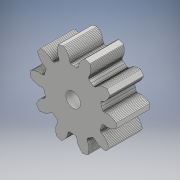
# Autodesk Inventor part: Engranajes PEQUENO final 2017
Saved by Autodesk Inventor 2019 (Build 230136000, 136)
## iProperties
Created: 2017-09-25
Part Number: Engranajes PEQUENO final 2017
Material: Generic
Document SubType Name: Modeling
Designer: ANDRES
Density: 1 g/cm^3
Appearance: Default
Author: ANDRES
## iProperties of the stored document Engranajes PEQUENO final 2017_3DPrint.ipt
Created: 2017-09-25
Part Number: Engranajes PEQUENO final 2017_3DPrint
Material: Generic
Document SubType Name: Modeling
Designer: ANDRES
Density: 1 g/cm^3
Appearance: Default
Author: ANDRES
Autodesk Inventor part; units mm, degrees
ref_plane "YZ Plane" through (0, 0, 0) normal (1, 0, 0) x (0, 1, 0)
ref_plane "XZ Plane" through (0, 0, 0) normal (0, 1, 0) x (-1, 0, 0)
ref_plane "XY Plane" through (0, 0, 0) normal (0, 0, 1) x (1, 0, 0)
sketch "Sketch1" plane through (0, 0, 0) normal (0, 1, 0) x (-1, 0, 0)
  line L0 (1.2686, 3.1496) -> (1.234, 3.2065)
  line L1 (1.234, 3.2065) -> (1.2093, 3.2258)
  line L2 (1.2093, 3.2258) -> (1.1862, 3.2384)
  line L3 (1.1862, 3.2384) -> (1.1641, 3.2475)
  line L4 (1.1641, 3.2475) -> (1.1425, 3.2542)
  line L5 (1.1425, 3.2542) -> (1.1214, 3.259)
  line L6 (1.1214, 3.259) -> (1.08, 3.2647)
  line L7 (1.08, 3.2647) -> (1.0396, 3.2662)
  line L8 (1.0396, 3.2662) -> (0.9998, 3.2645)
  line L9 (0.9998, 3.2645) -> (0.9218, 3.2535)
  line L10 (0.9218, 3.2535) -> (0.8454, 3.2341)
  line L11 (0.8454, 3.2341) -> (0.7662, 3.2294)
  line L12 (0.7662, 3.2294) -> (0.6848, 3.2361)
  line L13 (0.6848, 3.2361) -> (0.6022, 3.2499)
  line L14 (0.6022, 3.2499) -> (0.5189, 3.27)
  line L15 (0.5189, 3.27) -> (0.435, 3.2958)
  line L16 (0.435, 3.2958) -> (0.3507, 3.3269)
  line L17 (0.3507, 3.3269) -> (0.2664, 3.3631)
  line L18 (0.2664, 3.3631) -> (0.182, 3.4043)
  line L19 (0.182, 3.4043) -> (0.0978, 3.4503)
  line L20 (0.0978, 3.4503) -> (0.0141, 3.5011)
  line L21 (0.0141, 3.5011) -> (0.0024, 3.9651)
  line L22 (0.0024, 3.9651) -> (0.0835, 4.02)
  line L23 (0.0835, 4.02) -> (0.1653, 4.0702)
  line L24 (0.1653, 4.0702) -> (0.2474, 4.1155)
  line L25 (0.2474, 4.1155) -> (0.3299, 4.156)
  line L26 (0.3299, 4.156) -> (0.4125, 4.1913)
  line L27 (0.4125, 4.1913) -> (0.495, 4.2212)
  line L28 (0.495, 4.2212) -> (0.5772, 4.2455)
  line L29 (0.5772, 4.2455) -> (0.659, 4.2635)
  line L30 (0.659, 4.2635) -> (0.7399, 4.2742)
  line L31 (0.7399, 4.2742) -> (0.8193, 4.2735)
  line L32 (0.8193, 4.2735) -> (0.8965, 4.258)
  line L33 (0.8965, 4.258) -> (0.975, 4.2509)
  line L34 (0.975, 4.2509) -> (1.0148, 4.2512)
  line L35 (1.0148, 4.2512) -> (1.0551, 4.2547)
  line L36 (1.0551, 4.2547) -> (1.0962, 4.2625)
  line L37 (1.0962, 4.2625) -> (1.117, 4.2684)
  line L38 (1.117, 4.2684) -> (1.1382, 4.2761)
  line L39 (1.1382, 4.2761) -> (1.1599, 4.2863)
  line L40 (1.1599, 4.2863) -> (1.1823, 4.3001)
  line L41 (1.1823, 4.3001) -> (1.206, 4.3206)
  line L42 (1.206, 4.3206) -> (1.2377, 4.3791)
  line L43 (1.2377, 4.3791) -> (1.2899, 4.5842)
  line L44 (1.2899, 4.5842) -> (1.3582, 4.7844)
  line L45 (1.3582, 4.7844) -> (1.3636, 4.8508)
  line L46 (1.3636, 4.8508) -> (1.355, 4.8809)
  line L47 (1.355, 4.8809) -> (1.3438, 4.9047)
  line L48 (1.3438, 4.9047) -> (1.3312, 4.9251)
  line L49 (1.3312, 4.9251) -> (1.3177, 4.9431)
  line L50 (1.3177, 4.9431) -> (1.3034, 4.9595)
  line L51 (1.3034, 4.9595) -> (1.2733, 4.9884)
  line L52 (1.2733, 4.9884) -> (1.2415, 5.0134)
  line L53 (1.2415, 5.0134) -> (1.2083, 5.0354)
  line L54 (1.2083, 5.0354) -> (1.1387, 5.0723)
  line L55 (1.1387, 5.0723) -> (1.0655, 5.1015)
  line L56 (1.0655, 5.1015) -> (0.9986, 5.1443)
  line L57 (0.9986, 5.1443) -> (0.9367, 5.1975)
  line L58 (0.9367, 5.1975) -> (0.8781, 5.2573)
  line L59 (0.8781, 5.2573) -> (0.8225, 5.3225)
  line L60 (0.8225, 5.3225) -> (0.7697, 5.3927)
  line L61 (0.7697, 5.3927) -> (0.7198, 5.4674)
  line L62 (0.7198, 5.4674) -> (0.6729, 5.5463)
  line L63 (0.6729, 5.5463) -> (0.6288, 5.6292)
  line L64 (0.6288, 5.6292) -> (0.5878, 5.7159)
  line L65 (0.5878, 5.7159) -> (0.5499, 5.8062)
  line L66 (0.5499, 5.8062) -> (0.8132, 6.1884)
  line L67 (0.8132, 6.1884) -> (0.9111, 6.1852)
  line L68 (0.9111, 6.1852) -> (1.0067, 6.1777)
  line L69 (1.0067, 6.1777) -> (1.0998, 6.1661)
  line L70 (1.0998, 6.1661) -> (1.1903, 6.1504)
  line L71 (1.1903, 6.1504) -> (1.2779, 6.1304)
  line L72 (1.2779, 6.1304) -> (1.3622, 6.1061)
  line L73 (1.3622, 6.1061) -> (1.443, 6.0774)
  line L74 (1.443, 6.0774) -> (1.5197, 6.0439)
  line L75 (1.5197, 6.0439) -> (1.5915, 6.005)
  line L76 (1.5915, 6.005) -> (1.6553, 5.9578)
  line L77 (1.6553, 5.9578) -> (1.7087, 5.8998)
  line L78 (1.7087, 5.8998) -> (1.768, 5.848)
  line L79 (1.768, 5.848) -> (1.8004, 5.8248)
  line L80 (1.8004, 5.8248) -> (1.8351, 5.804)
  line L81 (1.8351, 5.804) -> (1.8728, 5.7861)
  line L82 (1.8728, 5.7861) -> (1.8932, 5.7786)
  line L83 (1.8932, 5.7786) -> (1.9149, 5.7724)
  line L84 (1.9149, 5.7724) -> (1.9384, 5.7679)
  line L85 (1.9384, 5.7679) -> (1.9646, 5.766)
  line L86 (1.9646, 5.766) -> (1.9959, 5.7686)
  line L87 (1.9959, 5.7686) -> (2.0559, 5.7973)
  line L88 (2.0559, 5.7973) -> (2.2187, 5.9324)
  line L89 (2.2187, 5.9324) -> (2.3916, 6.0542)
  line L90 (2.3916, 6.0542) -> (2.435, 6.1047)
  line L91 (2.435, 6.1047) -> (2.4457, 6.1342)
  line L92 (2.4457, 6.1342) -> (2.4506, 6.1601)
  line L93 (2.4506, 6.1601) -> (2.4524, 6.1839)
  line L94 (2.4524, 6.1839) -> (2.4521, 6.2065)
  line L95 (2.4521, 6.2065) -> (2.4502, 6.2281)
  line L96 (2.4502, 6.2281) -> (2.4428, 6.2692)
  line L97 (2.4428, 6.2692) -> (2.4318, 6.3081)
  line L98 (2.4318, 6.3081) -> (2.4177, 6.3454)
  line L99 (2.4177, 6.3454) -> (2.3831, 6.4162)
  line L100 (2.3831, 6.4162) -> (2.3411, 6.4828)
  line L101 (2.3411, 6.4828) -> (2.3122, 6.5568)
  line L102 (2.3122, 6.5568) -> (2.2933, 6.6362)
  line L103 (2.2933, 6.6362) -> (2.281, 6.719)
  line L104 (2.281, 6.719) -> (2.2743, 6.8045)
  line L105 (2.2743, 6.8045) -> (2.2728, 6.8923)
  line L106 (2.2728, 6.8923) -> (2.2764, 6.982)
  line L107 (2.2764, 6.982) -> (2.2848, 7.0734)
  line L108 (2.2848, 7.0734) -> (2.2979, 7.1664)
  line L109 (2.2979, 7.1664) -> (2.3155, 7.2606)
  line L110 (2.3155, 7.2606) -> (2.3379, 7.356)
  line L111 (2.3379, 7.356) -> (2.7756, 7.5106)
  line L112 (2.7756, 7.5106) -> (2.8529, 7.4504)
  line L113 (2.8529, 7.4504) -> (2.9259, 7.3882)
  line L114 (2.9259, 7.3882) -> (2.9944, 7.3241)
  line L115 (2.9944, 7.3241) -> (3.0584, 7.2582)
  line L116 (3.0584, 7.2582) -> (3.1175, 7.1906)
  line L117 (3.1175, 7.1906) -> (3.1715, 7.1214)
  line L118 (3.1715, 7.1214) -> (3.22, 7.0507)
  line L119 (3.22, 7.0507) -> (3.2624, 6.9785)
  line L120 (3.2624, 6.9785) -> (3.2976, 6.9048)
  line L121 (3.2976, 6.9048) -> (3.3215, 6.8291)
  line L122 (3.3215, 6.8291) -> (3.3307, 6.7508)
  line L123 (3.3307, 6.7508) -> (3.3482, 6.674)
  line L124 (3.3482, 6.674) -> (3.3608, 6.6362)
  line L125 (3.3608, 6.6362) -> (3.3766, 6.599)
  line L126 (3.3766, 6.599) -> (3.3966, 6.5624)
  line L127 (3.3966, 6.5624) -> (3.4087, 6.5443)
  line L128 (3.4087, 6.5443) -> (3.4226, 6.5267)
  line L129 (3.4226, 6.5267) -> (3.439, 6.5092)
  line L130 (3.439, 6.5092) -> (3.459, 6.4922)
  line L131 (3.459, 6.4922) -> (3.4859, 6.476)
  line L132 (3.4859, 6.476) -> (3.5513, 6.4639)
  line L133 (3.5513, 6.4639) -> (3.7625, 6.4776)
  line L134 (3.7625, 6.4776) -> (3.974, 6.4746)
  line L135 (3.974, 6.4746) -> (4.0388, 6.49)
  line L136 (4.0388, 6.49) -> (4.0648, 6.5075)
  line L137 (4.0648, 6.5075) -> (4.084, 6.5255)
  line L138 (4.084, 6.5255) -> (4.0994, 6.5438)
  line L139 (4.0994, 6.5438) -> (4.1124, 6.5622)
  line L140 (4.1124, 6.5622) -> (4.1236, 6.5808)
  line L141 (4.1236, 6.5808) -> (4.1417, 6.6184)
  line L142 (4.1417, 6.6184) -> (4.1557, 6.6564)
  line L143 (4.1557, 6.6564) -> (4.1664, 6.6948)
  line L144 (4.1664, 6.6948) -> (4.18, 6.7724)
  line L145 (4.18, 6.7724) -> (4.1851, 6.851)
  line L146 (4.1851, 6.851) -> (4.2052, 6.9278)
  line L147 (4.2052, 6.9278) -> (4.2366, 7.0032)
  line L148 (4.2366, 7.0032) -> (4.2753, 7.0774)
  line L149 (4.2753, 7.0774) -> (4.3201, 7.1504)
  line L150 (4.3201, 7.1504) -> (4.3705, 7.2223)
  line L151 (4.3705, 7.2223) -> (4.4262, 7.2928)
  line L152 (4.4262, 7.2928) -> (4.4867, 7.3619)
  line L153 (4.4867, 7.3619) -> (4.5519, 7.4295)
  line L154 (4.5519, 7.4295) -> (4.6217, 7.4952)
  line L155 (4.6217, 7.4952) -> (4.6958, 7.5591)
  line L156 (4.6958, 7.5591) -> (5.1408, 7.4269)
  line L157 (5.1408, 7.4269) -> (5.1679, 7.3327)
  line L158 (5.1679, 7.3327) -> (5.1904, 7.2395)
  line L159 (5.1904, 7.2395) -> (5.208, 7.1473)
  line L160 (5.208, 7.1473) -> (5.221, 7.0564)
  line L161 (5.221, 7.0564) -> (5.2292, 6.967)
  line L162 (5.2292, 6.967) -> (5.2321, 6.8792)
  line L163 (5.2321, 6.8792) -> (5.2298, 6.7935)
  line L164 (5.2298, 6.7935) -> (5.2216, 6.7102)
  line L165 (5.2216, 6.7102) -> (5.2068, 6.63)
  line L166 (5.2068, 6.63) -> (5.1816, 6.5546)
  line L167 (5.1816, 6.5546) -> (5.143, 6.486)
  line L168 (5.143, 6.486) -> (5.112, 6.4136)
  line L169 (5.112, 6.4136) -> (5.1001, 6.3756)
  line L170 (5.1001, 6.3756) -> (5.091, 6.3362)
  line L171 (5.091, 6.3362) -> (5.0857, 6.2948)
  line L172 (5.0857, 6.2948) -> (5.0849, 6.2731)
  line L173 (5.0849, 6.2731) -> (5.0857, 6.2505)
  line L174 (5.0857, 6.2505) -> (5.0887, 6.2268)
  line L175 (5.0887, 6.2268) -> (5.0949, 6.2012)
  line L176 (5.0949, 6.2012) -> (5.1071, 6.1723)
  line L177 (5.1071, 6.1723) -> (5.1529, 6.124)
  line L178 (5.1529, 6.124) -> (5.3318, 6.0111)
  line L179 (5.3318, 6.0111) -> (5.5011, 5.8842)
  line L180 (5.5011, 5.8842) -> (5.5625, 5.8587)
  line L181 (5.5625, 5.8587) -> (5.5939, 5.8576)
  line L182 (5.5939, 5.8576) -> (5.62, 5.8609)
  line L183 (5.62, 5.8609) -> (5.6433, 5.8666)
  line L184 (5.6433, 5.8666) -> (5.6646, 5.8738)
  line L185 (5.6646, 5.8738) -> (5.6846, 5.8823)
  line L186 (5.6846, 5.8823) -> (5.7213, 5.9021)
  line L187 (5.7213, 5.9021) -> (5.755, 5.9246)
  line L188 (5.755, 5.9246) -> (5.7861, 5.9494)
  line L189 (5.7861, 5.9494) -> (5.8428, 6.0042)
  line L190 (5.8428, 6.0042) -> (5.8932, 6.0647)
  line L191 (5.8932, 6.0647) -> (5.9545, 6.1151)
  line L192 (5.9545, 6.1151) -> (6.0243, 6.1575)
  line L193 (6.0243, 6.1575) -> (6.0992, 6.1948)
  line L194 (6.0992, 6.1948) -> (6.1784, 6.2277)
  line L195 (6.1784, 6.2277) -> (6.2615, 6.2562)
  line L196 (6.2615, 6.2562) -> (6.3479, 6.2805)
  line L197 (6.3479, 6.2805) -> (6.4375, 6.3008)
  line L198 (6.4375, 6.3008) -> (6.5299, 6.3171)
  line L199 (6.5299, 6.3171) -> (6.6251, 6.3293)
  line L200 (6.6251, 6.3293) -> (6.7227, 6.3375)
  line L201 (6.7227, 6.3375) -> (7.0048, 5.969)
  line L202 (7.0048, 5.969) -> (6.9715, 5.8769)
  line L203 (6.9715, 5.8769) -> (6.935, 5.7883)
  line L204 (6.935, 5.7883) -> (6.8951, 5.7033)
  line L205 (6.8951, 5.7033) -> (6.8522, 5.6221)
  line L206 (6.8522, 5.6221) -> (6.8061, 5.5449)
  line L207 (6.8061, 5.5449) -> (6.757, 5.4722)
  line L208 (6.757, 5.4722) -> (6.7047, 5.4043)
  line L209 (6.7047, 5.4043) -> (6.6492, 5.3416)
  line L210 (6.6492, 5.3416) -> (6.59, 5.2854)
  line L211 (6.59, 5.2854) -> (6.5253, 5.2393)
  line L212 (6.5253, 5.2393) -> (6.4538, 5.2064)
  line L213 (6.4538, 5.2064) -> (6.3862, 5.1661)
  line L214 (6.3862, 5.1661) -> (6.3541, 5.1424)
  line L215 (6.3541, 5.1424) -> (6.3236, 5.1158)
  line L216 (6.3236, 5.1158) -> (6.295, 5.0855)
  line L217 (6.295, 5.0855) -> (6.2816, 5.0684)
  line L218 (6.2816, 5.0684) -> (6.269, 5.0497)
  line L219 (6.269, 5.0497) -> (6.2574, 5.0287)
  line L220 (6.2574, 5.0287) -> (6.2474, 5.0044)
  line L221 (6.2474, 5.0044) -> (6.2403, 4.9739)
  line L222 (6.2403, 4.9739) -> (6.249, 4.9079)
  line L223 (6.249, 4.9079) -> (6.3273, 4.7113)
  line L224 (6.3273, 4.7113) -> (6.3897, 4.5092)
  line L225 (6.3897, 4.5092) -> (6.4244, 4.4523)
  line L226 (6.4244, 4.4523) -> (6.4491, 4.433)
  line L227 (6.4491, 4.433) -> (6.4722, 4.4203)
  line L228 (6.4722, 4.4203) -> (6.4943, 4.4113)
  line L229 (6.4943, 4.4113) -> (6.5159, 4.4046)
  line L230 (6.5159, 4.4046) -> (6.537, 4.3997)
  line L231 (6.537, 4.3997) -> (6.5783, 4.3941)
  line L232 (6.5783, 4.3941) -> (6.6188, 4.3926)
  line L233 (6.6188, 4.3926) -> (6.6586, 4.3943)
  line L234 (6.6586, 4.3943) -> (6.7366, 4.4053)
  line L235 (6.7366, 4.4053) -> (6.8129, 4.4247)
  line L236 (6.8129, 4.4247) -> (6.8922, 4.4293)
  line L237 (6.8922, 4.4293) -> (6.9736, 4.4227)
  line L238 (6.9736, 4.4227) -> (7.0561, 4.4088)
  line L239 (7.0561, 4.4088) -> (7.1395, 4.3887)
  line L240 (7.1395, 4.3887) -> (7.2234, 4.363)
  line L241 (7.2234, 4.363) -> (7.3076, 4.3319)
  line L242 (7.3076, 4.3319) -> (7.392, 4.2956)
  line L243 (7.392, 4.2956) -> (7.4764, 4.2545)
  line L244 (7.4764, 4.2545) -> (7.5605, 4.2084)
  line L245 (7.5605, 4.2084) -> (7.6443, 4.1577)
  line L246 (7.6443, 4.1577) -> (7.656, 3.6937)
  line L247 (7.656, 3.6937) -> (7.5748, 3.639)
  line L248 (7.5748, 3.639) -> (7.4931, 3.5888)
  line L249 (7.4931, 3.5888) -> (7.4109, 3.5434)
  line L250 (7.4109, 3.5434) -> (7.3285, 3.503)
  line L251 (7.3285, 3.503) -> (7.2459, 3.4677)
  line L252 (7.2459, 3.4677) -> (7.1634, 3.4378)
  line L253 (7.1634, 3.4378) -> (7.0812, 3.4135)
  line L254 (7.0812, 3.4135) -> (6.9994, 3.3955)
  line L255 (6.9994, 3.3955) -> (6.9185, 3.3848)
  line L256 (6.9185, 3.3848) -> (6.8391, 3.3855)
  line L257 (6.8391, 3.3855) -> (6.7618, 3.401)
  line L258 (6.7618, 3.401) -> (6.6834, 3.4081)
  line L259 (6.6834, 3.4081) -> (6.6436, 3.4078)
  line L260 (6.6436, 3.4078) -> (6.6032, 3.4042)
  line L261 (6.6032, 3.4042) -> (6.5622, 3.3965)
  line L262 (6.5622, 3.3965) -> (6.5414, 3.3906)
  line L263 (6.5414, 3.3906) -> (6.5202, 3.3829)
  line L264 (6.5202, 3.3829) -> (6.4985, 3.3727)
  line L265 (6.4985, 3.3727) -> (6.4761, 3.3589)
  line L266 (6.4761, 3.3589) -> (6.4524, 3.3383)
  line L267 (6.4524, 3.3383) -> (6.4206, 3.2798)
  line L268 (6.4206, 3.2798) -> (6.3685, 3.0748)
  line L269 (6.3685, 3.0748) -> (6.3001, 2.8746)
  line L270 (6.3001, 2.8746) -> (6.2947, 2.8082)
  line L271 (6.2947, 2.8082) -> (6.3034, 2.7781)
  line L272 (6.3034, 2.7781) -> (6.3146, 2.7543)
  line L273 (6.3146, 2.7543) -> (6.3272, 2.7339)
  line L274 (6.3272, 2.7339) -> (6.3407, 2.7158)
  line L275 (6.3407, 2.7158) -> (6.355, 2.6995)
  line L276 (6.355, 2.6995) -> (6.3851, 2.6706)
  line L277 (6.3851, 2.6706) -> (6.4169, 2.6456)
  line L278 (6.4169, 2.6456) -> (6.4501, 2.6236)
  line L279 (6.4501, 2.6236) -> (6.5197, 2.5867)
  line L280 (6.5197, 2.5867) -> (6.5929, 2.5574)
  line L281 (6.5929, 2.5574) -> (6.6597, 2.5146)
  line L282 (6.6597, 2.5146) -> (6.7217, 2.4614)
  line L283 (6.7217, 2.4614) -> (6.7803, 2.4017)
  line L284 (6.7803, 2.4017) -> (6.8359, 2.3365)
  line L285 (6.8359, 2.3365) -> (6.8887, 2.2663)
  line L286 (6.8887, 2.2663) -> (6.9385, 2.1916)
  line L287 (6.9385, 2.1916) -> (6.9855, 2.1127)
  line L288 (6.9855, 2.1127) -> (7.0295, 2.0298)
  line L289 (7.0295, 2.0298) -> (7.0706, 1.9431)
  line L290 (7.0706, 1.9431) -> (7.1085, 1.8528)
  line L291 (7.1085, 1.8528) -> (6.8452, 1.4705)
  line L292 (6.8452, 1.4705) -> (6.7473, 1.4738)
  line L293 (6.7473, 1.4738) -> (6.6517, 1.4813)
  line L294 (6.6517, 1.4813) -> (6.5585, 1.4929)
  line L295 (6.5585, 1.4929) -> (6.4681, 1.5086)
  line L296 (6.4681, 1.5086) -> (6.3805, 1.5286)
  line L297 (6.3805, 1.5286) -> (6.2962, 1.5529)
  line L298 (6.2962, 1.5529) -> (6.2154, 1.5816)
  line L299 (6.2154, 1.5816) -> (6.1387, 1.6151)
  line L300 (6.1387, 1.6151) -> (6.0669, 1.654)
  line L301 (6.0669, 1.654) -> (6.0032, 1.7012)
  line L302 (6.0032, 1.7012) -> (5.9498, 1.7591)
  line L303 (5.9498, 1.7591) -> (5.8905, 1.811)
  line L304 (5.8905, 1.811) -> (5.8581, 1.8342)
  line L305 (5.8581, 1.8342) -> (5.8234, 1.855)
  line L306 (5.8234, 1.855) -> (5.7857, 1.8729)
  line L307 (5.7857, 1.8729) -> (5.7653, 1.8803)
  line L308 (5.7653, 1.8803) -> (5.7436, 1.8865)
  line L309 (5.7436, 1.8865) -> (5.7201, 1.891)
  line L310 (5.7201, 1.891) -> (5.6939, 1.893)
  line L311 (5.6939, 1.893) -> (5.6626, 1.8904)
  line L312 (5.6626, 1.8904) -> (5.6025, 1.8617)
  line L313 (5.6025, 1.8617) -> (5.4398, 1.7264)
  line L314 (5.4398, 1.7264) -> (5.2668, 1.6045)
  line L315 (5.2668, 1.6045) -> (5.2235, 1.554)
  line L316 (5.2235, 1.554) -> (5.2128, 1.5245)
  line L317 (5.2128, 1.5245) -> (5.2078, 1.4987)
  line L318 (5.2078, 1.4987) -> (5.2061, 1.4748)
  line L319 (5.2061, 1.4748) -> (5.2065, 1.4523)
  line L320 (5.2065, 1.4523) -> (5.2084, 1.4307)
  line L321 (5.2084, 1.4307) -> (5.2158, 1.3896)
  line L322 (5.2158, 1.3896) -> (5.2268, 1.3507)
  line L323 (5.2268, 1.3507) -> (5.2407, 1.3133)
  line L324 (5.2407, 1.3133) -> (5.2754, 1.2426)
  line L325 (5.2754, 1.2426) -> (5.3174, 1.1759)
  line L326 (5.3174, 1.1759) -> (5.3463, 1.102)
  line L327 (5.3463, 1.102) -> (5.3651, 1.0225)
  line L328 (5.3651, 1.0225) -> (5.3774, 0.9398)
  line L329 (5.3774, 0.9398) -> (5.3841, 0.8543)
  line L330 (5.3841, 0.8543) -> (5.3855, 0.7665)
  line L331 (5.3855, 0.7665) -> (5.3821, 0.6768)
  line L332 (5.3821, 0.6768) -> (5.3737, 0.5853)
  line L333 (5.3737, 0.5853) -> (5.3606, 0.4924)
  line L334 (5.3606, 0.4924) -> (5.3428, 0.3981)
  line L335 (5.3428, 0.3981) -> (5.3205, 0.3028)
  line L336 (5.3205, 0.3028) -> (4.8829, 0.1482)
  line L337 (4.8829, 0.1482) -> (4.8056, 0.2084)
  line L338 (4.8056, 0.2084) -> (4.7325, 0.2706)
  line L339 (4.7325, 0.2706) -> (4.6639, 0.3347)
  line L340 (4.6639, 0.3347) -> (4.6, 0.4006)
  line L341 (4.6, 0.4006) -> (4.5409, 0.4682)
  line L342 (4.5409, 0.4682) -> (4.487, 0.5374)
  line L343 (4.487, 0.5374) -> (4.4385, 0.6081)
  line L344 (4.4385, 0.6081) -> (4.3961, 0.6803)
  line L345 (4.3961, 0.6803) -> (4.3608, 0.754)
  line L346 (4.3608, 0.754) -> (4.3369, 0.8297)
  line L347 (4.3369, 0.8297) -> (4.3278, 0.9079)
  line L348 (4.3278, 0.9079) -> (4.3103, 0.9848)
  line L349 (4.3103, 0.9848) -> (4.2977, 1.0225)
  line L350 (4.2977, 1.0225) -> (4.2819, 1.0598)
  line L351 (4.2819, 1.0598) -> (4.2619, 1.0964)
  line L352 (4.2619, 1.0964) -> (4.2498, 1.1144)
  line L353 (4.2498, 1.1144) -> (4.2359, 1.1322)
  line L354 (4.2359, 1.1322) -> (4.2195, 1.1496)
  line L355 (4.2195, 1.1496) -> (4.1994, 1.1667)
  line L356 (4.1994, 1.1667) -> (4.1726, 1.1829)
  line L357 (4.1726, 1.1829) -> (4.1071, 1.195)
  line L358 (4.1071, 1.195) -> (3.896, 1.1812)
  line L359 (3.896, 1.1812) -> (3.6845, 1.1844)
  line L360 (3.6845, 1.1844) -> (3.6197, 1.169)
  line L361 (3.6197, 1.169) -> (3.5937, 1.1514)
  line L362 (3.5937, 1.1514) -> (3.5745, 1.1334)
  line L363 (3.5745, 1.1334) -> (3.559, 1.1152)
  line L364 (3.559, 1.1152) -> (3.546, 1.0967)
  line L365 (3.546, 1.0967) -> (3.5349, 1.0781)
  line L366 (3.5349, 1.0781) -> (3.5167, 1.0405)
  line L367 (3.5167, 1.0405) -> (3.5028, 1.0025)
  line L368 (3.5028, 1.0025) -> (3.4921, 0.9641)
  line L369 (3.4921, 0.9641) -> (3.4785, 0.8865)
  line L370 (3.4785, 0.8865) -> (3.4733, 0.8079)
  line L371 (3.4733, 0.8079) -> (3.4533, 0.7311)
  line L372 (3.4533, 0.7311) -> (3.4218, 0.6557)
  line L373 (3.4218, 0.6557) -> (3.3832, 0.5815)
  line L374 (3.3832, 0.5815) -> (3.3384, 0.5084)
  line L375 (3.3384, 0.5084) -> (3.2879, 0.4366)
  line L376 (3.2879, 0.4366) -> (3.2323, 0.3661)
  line L377 (3.2323, 0.3661) -> (3.1718, 0.297)
  line L378 (3.1718, 0.297) -> (3.1065, 0.2295)
  line L379 (3.1065, 0.2295) -> (3.0368, 0.1637)
  line L380 (3.0368, 0.1637) -> (2.9626, 0.0997)
  line L381 (2.9626, 0.0997) -> (2.5177, 0.2319)
  line L382 (2.5177, 0.2319) -> (2.4906, 0.326)
  line L383 (2.4906, 0.326) -> (2.4681, 0.4193)
  line L384 (2.4681, 0.4193) -> (2.4503, 0.5114)
  line L385 (2.4503, 0.5114) -> (2.4374, 0.6024)
  line L386 (2.4374, 0.6024) -> (2.4292, 0.6918)
  line L387 (2.4292, 0.6918) -> (2.4262, 0.7795)
  line L388 (2.4262, 0.7795) -> (2.4286, 0.8652)
  line L389 (2.4286, 0.8652) -> (2.4367, 0.9485)
  line L390 (2.4367, 0.9485) -> (2.4516, 1.0288)
  line L391 (2.4516, 1.0288) -> (2.4767, 1.1041)
  line L392 (2.4767, 1.1041) -> (2.5153, 1.1728)
  line L393 (2.5153, 1.1728) -> (2.5463, 1.2452)
  line L394 (2.5463, 1.2452) -> (2.5583, 1.2832)
  line L395 (2.5583, 1.2832) -> (2.5674, 1.3226)
  line L396 (2.5674, 1.3226) -> (2.5727, 1.364)
  line L397 (2.5727, 1.364) -> (2.5735, 1.3857)
  line L398 (2.5735, 1.3857) -> (2.5727, 1.4082)
  line L399 (2.5727, 1.4082) -> (2.5697, 1.432)
  line L400 (2.5697, 1.432) -> (2.5635, 1.4575)
  line L401 (2.5635, 1.4575) -> (2.5513, 1.4865)
  line L402 (2.5513, 1.4865) -> (2.5055, 1.5347)
  line L403 (2.5055, 1.5347) -> (2.3266, 1.6477)
  line L404 (2.3266, 1.6477) -> (2.1573, 1.7745)
  line L405 (2.1573, 1.7745) -> (2.0958, 1.8001)
  line L406 (2.0958, 1.8001) -> (2.0645, 1.8012)
  line L407 (2.0645, 1.8012) -> (2.0384, 1.7979)
  line L408 (2.0384, 1.7979) -> (2.0151, 1.7922)
  line L409 (2.0151, 1.7922) -> (1.9938, 1.7849)
  line L410 (1.9938, 1.7849) -> (1.9738, 1.7764)
  line L411 (1.9738, 1.7764) -> (1.937, 1.7567)
  line L412 (1.937, 1.7567) -> (1.9034, 1.7342)
  line L413 (1.9034, 1.7342) -> (1.8722, 1.7094)
  line L414 (1.8722, 1.7094) -> (1.8156, 1.6546)
  line L415 (1.8156, 1.6546) -> (1.7652, 1.5941)
  line L416 (1.7652, 1.5941) -> (1.7038, 1.5436)
  line L417 (1.7038, 1.5436) -> (1.6341, 1.5011)
  line L418 (1.6341, 1.5011) -> (1.5592, 1.4638)
  line L419 (1.5592, 1.4638) -> (1.4799, 1.4311)
  line L420 (1.4799, 1.4311) -> (1.3969, 1.4026)
  line L421 (1.3969, 1.4026) -> (1.3105, 1.3783)
  line L422 (1.3105, 1.3783) -> (1.2209, 1.358)
  line L423 (1.2209, 1.358) -> (1.1284, 1.3417)
  line L424 (1.1284, 1.3417) -> (1.0333, 1.3294)
  line L425 (1.0333, 1.3294) -> (0.9357, 1.3212)
  line L426 (0.9357, 1.3212) -> (0.6535, 1.6897)
  line L427 (0.6535, 1.6897) -> (0.6869, 1.7818)
  line L428 (0.6869, 1.7818) -> (0.7234, 1.8705)
  line L429 (0.7234, 1.8705) -> (0.7632, 1.9555)
  line L430 (0.7632, 1.9555) -> (0.8062, 2.0367)
  line L431 (0.8062, 2.0367) -> (0.8522, 2.1137)
  line L432 (0.8522, 2.1137) -> (0.9014, 2.1865)
  line L433 (0.9014, 2.1865) -> (0.9537, 2.2544)
  line L434 (0.9537, 2.2544) -> (1.0092, 2.317)
  line L435 (1.0092, 2.317) -> (1.0684, 2.3733)
  line L436 (1.0684, 2.3733) -> (1.133, 2.4195)
  line L437 (1.133, 2.4195) -> (1.2045, 2.4524)
  line L438 (1.2045, 2.4524) -> (1.2722, 2.4927)
  line L439 (1.2722, 2.4927) -> (1.3042, 2.5164)
  line L440 (1.3042, 2.5164) -> (1.3348, 2.5429)
  line L441 (1.3348, 2.5429) -> (1.3634, 2.5733)
  line L442 (1.3634, 2.5733) -> (1.3768, 2.5903)
  line L443 (1.3768, 2.5903) -> (1.3894, 2.6091)
  line L444 (1.3894, 2.6091) -> (1.4009, 2.63)
  line L445 (1.4009, 2.63) -> (1.4109, 2.6544)
  line L446 (1.4109, 2.6544) -> (1.4181, 2.6849)
  line L447 (1.4181, 2.6849) -> (1.4094, 2.7509)
  line L448 (1.4094, 2.7509) -> (1.331, 2.9475)
  line L449 (1.331, 2.9475) -> (1.2686, 3.1496)
  circle A0 centre (3.8291, 3.8291) radius 0.65
  point P0 (0, 0)
  dimension "d2" = 1.3
  constraints: 900 end point, 79 parallel, 10 perpendicular, 1 centre point
  measures "d2" diameter of A0
extrude "Extrusion2" add sketch "Sketch1" along normal blind 3
body "Solid2"
